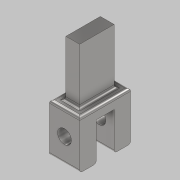
# Autodesk Inventor part: support_sandwichPlate
Saved by Autodesk Inventor 2021 (Build 250183000, 183)
## iProperties
Created: 2021-05-11
Part Number: support_sandwichPlate
Material: Steel, Carbon
Document SubType Name: Modeling
Designer: Watchdog
Density: 7.85 g/cm^3
Appearance: Semi-Polished
Author: Watchdog
Autodesk Inventor part; units mm, degrees
ref_plane "YZ Plane" through (0, 0, 0) normal (1, 0, 0) x (0, 1, 0)
ref_plane "XZ Plane" through (0, 0, 0) normal (0, 1, 0) x (-1, 0, 0)
ref_plane "XY Plane" through (0, 0, 0) normal (0, 0, 1) x (1, 0, 0)
sketch "Sketch1" plane through (0, 0, 0) normal (1, 0, 0) x (0, 1, 0)
  line L0 (20, 12.5) -> (-20, 12.5)
  line L1 (-20, 12.5) -> (-20, -12.5)
  line L2 (-20, -12.5) -> (20, -12.5)
  line L3 (20, -12.5) -> (20, 12.5)
  point P0 (0, 0)
  dimension "d0" = 25
  dimension "d1" = 40
  dimension "d2" = 20
  dimension "d3" = 12.5
  constraints: 8 end point, 2 parallel, 1 horizontal, 1 perpendicular
  measures "d0" distance of L2.end L0.start
  measures "d1" distance of L0.start L0.end
  measures "d2" distance from line of point (0, 0) L3
  measures "d3" distance from line of point (0, 0) L0
extrude "sandwich_plate" add sketch "Sketch1" along normal blind 10
sketch "Sketch2" plane through (0, -20, -12.5) normal (0, -1, 0) x (1, 0, 0)
  line L0 (16, -6) -> (-6, -6)
  line L1 (-6, -6) -> (-6, 31)
  line L2 (-6, 31) -> (16, 31)
  line L3 (16, 31) -> (16, -6)
  line L4 (0, 25) -> (10, 25) projected
  line L5 (0, 0) -> (10, 0) projected
  line L6 (10, 25) -> (10, 0) projected
  line L7 (0, 25) -> (0, 0) projected
  point P0 (0, 12.5)
  dimension "d9" = 6
  dimension "d10" = 6
  dimension "d11" = 6
  dimension "d12" = 6
  constraints: 8 end point
  measures "d9" distance between parallel lines of L4 L2
  measures "d10" distance between parallel lines of L0 L5
  measures "d11" distance between parallel lines of L3 L6
  measures "d12" distance between parallel lines of L7 L1
extrude "clamp_length" add sketch "Sketch2" along normal blind 35 contours L0 L1 L2 L3 | L4 L6 L5 L7
sketch "Sketch3" plane through (16, -20, 18.5) normal (1, 0, 0) x (0, 0, -1)
  line L0 (0, -35) -> (37, -35) projected
  line L1 (12, -35) -> (25, -35)
  line L2 (25, -35) -> (25, -7.5)
  line L3 (25, -7.5) -> (12, -7.5)
  line L4 (12, -7.5) -> (12, -35)
  line L5 (37, 0) -> (0, 0) projected
  line L6 (0, 0) -> (0, -35) projected
  line L7 (37, 0) -> (37, -35) projected
  point P0 (18.5, 20)
  dimension "d14" = 7.5
  dimension "d15" = 12
  dimension "d16" = 12
  constraints: 8 end point, 2 parallel, 1 horizontal, 1 perpendicular, 1 point on line
  measures "d14" distance between parallel lines of L5 L3
  measures "d15" distance between parallel lines of L6 L4
  measures "d16" distance between parallel lines of L7 L2
extrude "slot" cut sketch "Sketch3" against normal through all contours L4 L3 L2 L0
fillet "Fillet1" radius 2 12 edges at (5, -20, 12.5) (10, -20, 0) (0, -20, 0) (5, -20, -12.5) (16, -20, 0) (5, -20, 18.5) (-6, -20, 0) (5, -20, -18.5) (5, -55, 6.5) (5, -55, -6.5) (5, -55, 18.5) (5, -55, -18.5)
sketch "Sketch4" plane through (-6, -55, 18.5) normal (0, 0, 1) x (1, 0, 0)
  line L0 (22, 33) -> (22, 0) projected
  line L1 (22, 0) -> (0, 0) projected
  point P0 (6, 55)
  point P1 (11, 17.5)
  dimension "d20" = 11
  dimension "d21" = 17.5
  measures "d20" distance from line of L0 point (11, 17.5)
  measures "d21" distance from line of L1 point (11, 17.5)
hole "Hole1" at (5, -37.5, 18.5) direction (0, 0, -1) diameter 10 end through all
equation "\"d2\" = 0.5 * d1"
equation "\"d3\" = 0.5 * d0"
equation "\"d10\" = d9"
equation "\"d11\" = d9"
equation "\"d12\" = d11"
equation "\"d16\" = d15"
equation "\"d21\" = 0.5 * d7"
equation "\"d7\" = 35"
body "Solid1"
